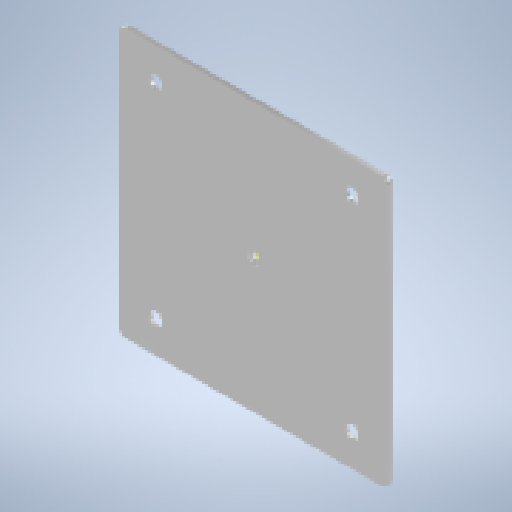
# Autodesk Inventor part: Plate
Saved by Autodesk Inventor 2025.3 (Build 293356000, 356)
## iProperties
Created: 2025-10-10
Part Number: Plate
Material: Aluminum 6061
Document SubType Name: Modeling
Designer: Haggag
Density: 2.7 g/cm^3
Appearance: Aluminum - Flat
Author: Haggag
Autodesk Inventor part; units mm, degrees
ref_plane "YZ Plane" through (0, 0, 0) normal (1, 0, 0) x (0, 1, 0)
ref_plane "XZ Plane" through (0, 0, 0) normal (0, 1, 0) x (-1, 0, 0)
ref_plane "XY Plane" through (0, 0, 0) normal (0, 0, 1) x (1, 0, 0)
sketch "Sketch1" plane through (0, 0, 0) normal (0, 0, 1) x (1, 0, 0)
  line L0 (100, 100) -> (-100, 100)
  line L1 (-100, 100) -> (-100, -100)
  line L2 (-100, -100) -> (100, -100)
  line L3 (100, -100) -> (100, 100)
  line L4 (100, 100) -> (-100, -100) construction
  line L5 (-100, 100) -> (100, -100) construction
  point P0 (0, 0)
  dimension "d0" = 200
  dimension "d1" = 200
  constraints: 12 end point, 2 midpoint, 2 parallel, 1 horizontal, 1 perpendicular
  measures "d0" distance of L2.end L1.end
  measures "d1" distance of L1.end L0.end
extrude "Extrusion1" add sketch "Sketch1" along normal blind 3
fillet "Fillet1" radius 5 4 edges at (100, 100, 1.5) (-100, 100, 1.5) (100, -100, 1.5) (-100, -100, 1.5)
sketch "Sketch2" plane through (0, 0, 3) normal (0, 0, 1) x (1, 0, 0)
  circle A0 centre (0, 0) radius 2.55
  dimension "d5" = 5.1
  constraints: 1 centre point, 1 coincident
  measures "d5" diameter of A0
extrude "Extrusion2" cut sketch "Sketch2" against normal blind 10
sketch "Sketch3" plane through (0, 0, 3) normal (0, 0, 1) x (1, 0, 0)
  circle A0 centre (0, 0) radius 4.75
  dimension "d10" = 9.5
  constraints: 1 centre point
  measures "d10" diameter of A0
extrude "Extrusion3" cut sketch "Sketch3" against normal blind 0.7
sketch "Sketch4" plane through (0, 0, 0) normal (0, 0, -1) x (-1, 0, 0)
  point P0 (0, 0)
sketch "Sketch5" plane through (0, 0, 0) normal (0, 0, -1) x (-1, 0, 0)
  point P0 (0, 0)
sketch "Sketch6" plane through (0, 0, 0) normal (0, 0, -1) x (-1, 0, 0)
  circle A0 centre (-72.965, 76.2324) radius 6
  line L0 (-93.7439, 99.9999) -> (-93.7439, -0.0001)
  line L1 (-93.7439, -0.0001) -> (78.7368, -0.0001)
  circle A1 centre (-72.965, -76.2325) radius 6
  line L2 (95, -100) -> (-95, -100) projected
  line L3 (0, -100) -> (0, 48.6306)
  circle A2 centre (72.965, 76.2324) radius 6
  circle A3 centre (72.965, -76.2325) radius 6
  point P0 (0, 0)
  point P1 (-93.7439, 89.8675)
  point P2 (-93.7439, 85.1564)
  dimension "d11" = 12
  dimension "d13" = 100
  constraints: 6 end point, 4 centre point, 3 symmetric about line, 2 vertical, 1 midpoint, 1 perpendicular, 3 other
  measures "d11" diameter of A0
  measures "d13" distance of L0.start L0.end
extrude "Extrusion4" cut sketch "Sketch6" against normal blind 10
sketch "Sketch7" plane through (0, 0, 3) normal (0, 0, 1) x (1, 0, 0)
  circle A0 centre (-72.965, 76.2324) radius 5
  circle A1 centre (0, 0) radius 2.55 projected
  line L0 (0, 0) -> (0, 15.1871)
  circle A2 centre (0, 0) radius 4.75 projected
  line L1 (0, 0) -> (12.7687, 0)
  circle A3 centre (72.965, 76.2324) radius 5
  circle A4 centre (-72.965, -76.2324) radius 5
  circle A5 centre (72.965, -76.2324) radius 5
  circle A6 centre (-72.965, 76.2324) radius 6
  circle A7 centre (72.965, 76.2324) radius 6
  circle A8 centre (-72.965, -76.2324) radius 5.9998
  circle A9 centre (72.965, -76.2324) radius 5.9998
  circle A10 centre (-72.965, 76.2324) radius 6
  dimension "d16" = 10
  constraints: 9 centre point, 6 coincident, 4 end point, 3 symmetric about line, 1 concentric, 1 horizontal, 1 vertical, 3 other
  measures "d16" diameter of A0
extrude "Extrusion5" add sketch "Sketch7" against normal blind 1 contours A6 | A7 | A8 | A9
sketch "Sketch8" plane through (0, 0, 0) normal (0, 0, -1) x (-1, 0, 0)
  circle A0 centre (0, 0) radius 4.24
  dimension "d19" = 8.48
  constraints: 1 centre point, 1 coincident
  measures "d19" diameter of A0
extrude "Extrusion6" cut sketch "Sketch8" against normal blind 0.5
body "Solid1"
